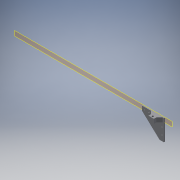
# Autodesk Inventor part: Bed Bracket
Saved by Autodesk Inventor 2016 (Build 200138000, 138)
## iProperties
Created: 2016-05-26
Part Number: Bed Bracket
Material: Generic
Document SubType Name: Modeling
Designer: Scott
Density: 1 g/cm^3
Appearance: Default
Author: Scott
Autodesk Inventor part; units mm, degrees
ref_plane "YZ Plane" through (0, 0, 0) normal (1, 0, 0) x (0, 1, 0)
ref_plane "XZ Plane" through (0, 0, 0) normal (0, 1, 0) x (-1, 0, 0)
ref_plane "XY Plane" through (0, 0, 0) normal (0, 0, 1) x (1, 0, 0)
ref_plane "Work Plane1" through (0, 0, 0) normal (0, 0, 1) x (1, 0, 0)
sketch "Sketch1" plane through (0, 0, 0) normal (0, 0, 1) x (1, 0, 0)
  line L0 (0, 0) -> (304.8, 0)
  line L1 (304.8, 0) -> (292.1, 0)
  line L2 (-330.2, 20) -> (330.2, 20) projected
  line L3 (-330.2, 0) -> (-330.2, 20) projected
  line L4 (330.2, 0) -> (-330.2, 0) projected
  line L5 (330.2, 20) -> (330.2, 0) projected
  line L6 (292.1, 0) -> (292.1, 10)
  line L7 (330.6445, 0) -> (253.5555, 0)
  line L8 (253.5555, 0) -> (253.5555, 20)
  line L9 (253.5555, 20) -> (330.6445, 20)
  line L10 (330.6445, 20) -> (330.6445, 0)
  line L11 (330.6445, 0) -> (253.5555, 20) construction
  line L12 (253.5555, 0) -> (330.6445, 20) construction
  line L13 (330.6445, 0) -> (330.6445, -76.2)
  line L14 (330.6445, 0) -> (406.8445, 0) construction
  line L15 (330.6445, -76.2) -> (310.8751, -76.2)
  line L16 (330.6445, 20) -> (229.0445, 20)
  line L17 (229.0445, 20) -> (229.0445, 0)
  line L18 (229.0445, 0) -> (310.8751, -76.2)
  line L19 (310.8751, -76.2) -> (310.8751, 0)
  dimension "d0" = 304.8
  dimension "d1" = 12.7
  dimension "d2" = 76.2
  dimension "d3" = 90
  dimension "d4" = 101.6
  constraints: 32 end point, 5 point on line, 4 parallel, 3 horizontal, 3 perpendicular, 2 midpoint, 2 vertical
  measures "d0" distance of L0.start L0.end
  measures "d1" distance of L0.end L1.end
  measures "d2" distance of L7.start L13.end
  measures "d3" angle of L13 L14
  measures "d4" distance of L9.end L16.end
extrude "Extrusion1" add sketch "Sketch1" along normal blind 5.08 contours L17 L2 L8 L0 | L0 L4 L19 L18 | L8 L2 L5 L4 L0 | L19 L4 L7 L13 L15 | L9 L10 L7 L5
sketch "Sketch2" plane through (0, 0, 5.08) normal (0, 0, 1) x (1, 0, 0)
  line L0 (310.2, -876.3) -> (310.2, 0) projected
  line L1 (310.2, 0) -> (297.5, 0)
  line L2 (297.5, 0) -> (297.5, 10)
  line L3 (284.8, 20) -> (310.2, 20)
  line L4 (310.2, 20) -> (310.2, 0)
  line L5 (310.2, 0) -> (284.8, 0)
  line L6 (284.8, 0) -> (284.8, 20)
  line L7 (284.8, 20) -> (310.2, 0) construction
  line L8 (310.2, 20) -> (284.8, 0) construction
  point P0 (0, 0)
  dimension "d7" = 12.7
  dimension "d8" = 10
  dimension "d9" = 90
  constraints: 16 end point, 2 horizontal, 2 midpoint, 2 parallel, 2 perpendicular
  measures "d7" distance of L0.end L1.end
  measures "d8" distance of L1.end L2.end
  measures "d9" angle of L1 L2
extrude "Extrusion2" add sketch "Sketch2" along normal blind 25.4
sketch "Sketch3" plane through (229.0445, 20, 0) normal (0, 1, 0) x (1, 0, 0)
  line L0 (101.6, 0) -> (0, 0) projected
  line L1 (0, 0) -> (0, -5.08) projected
  line L2 (55.7555, -5.08) -> (0, -5.08) projected
  line L3 (55.7555, -5.08) -> (55.7555, -30.48) projected
  line L4 (81.1555, -30.48) -> (55.7555, -30.48) projected
  line L5 (81.1555, -5.08) -> (81.1555, -30.48) projected
  line L6 (101.6, -5.08) -> (81.1555, -5.08) projected
  line L7 (101.6, 0) -> (101.6, -5.08) projected
  circle A0 centre (68.4555, -22.86) radius 4
  point P0 (-229.0445, 0)
  dimension "d12" = 8
  dimension "d13" = 7.62
  constraints: 1 centre point
  measures "d12" diameter of A0
  measures "d13" distance from line of L4 A0.centre
extrude "Extrusion3" cut sketch "Sketch3" against normal blind 101.6 contours A0
chamfer "Chamfer1" distance 14.2875 angle 45 2 edges at (284.8, 10, 5.08) (310.2, 10, 5.08)
sketch "Sketch4" plane through (0, 0, 5.08) normal (0, 0, 1) x (1, 0, 0)
  line L0 (324.4875, 0) -> (324.4875, 20) projected
  line L1 (324.4875, 0) -> (270.5125, 0) projected
  line L2 (270.5125, 20) -> (270.5125, 0) projected
  line L3 (270.5125, 20) -> (229.0445, 20) projected
  line L4 (229.0445, 20) -> (229.0445, 0) projected
  line L5 (229.0445, 0) -> (310.8751, -76.2) projected
  line L6 (310.8751, -76.2) -> (330.6445, -76.2) projected
  line L7 (330.6445, -76.2) -> (330.6445, 20) projected
  line L8 (330.6445, 20) -> (324.4875, 20) projected
  line L9 (330.2, 0) -> (330.2, -876.3) projected
  line L10 (310.2, 0) -> (330.2, 0) projected
  line L11 (310.2, -876.3) -> (310.2, 0) projected
  line L12 (330.2, -876.3) -> (310.2, -876.3) projected
  line L13 (324.4875, 0) -> (324.4875, 20) projected
  line L14 (324.4875, 0) -> (270.5125, 0) projected
  line L15 (270.5125, 20) -> (270.5125, 0) projected
  line L16 (270.5125, 20) -> (229.0445, 20) projected
  line L17 (229.0445, 20) -> (229.0445, 0) projected
  line L18 (229.0445, 0) -> (310.8751, -76.2) projected
  line L19 (310.8751, -76.2) -> (330.6445, -76.2) projected
  line L20 (330.6445, -76.2) -> (330.6445, 20) projected
  line L21 (330.6445, 20) -> (324.4875, 20) projected
  line L22 (330.2, 0) -> (-330.2, 0) projected
  circle A0 centre (320.7598, -50.8) radius 2.5
  circle A1 centre (320.7598, -19.05) radius 2.5
  circle A2 centre (241.7445, 10) radius 2.5
  circle A3 centre (260.7945, 10) radius 2.5
  point P0 (0, 0)
  dimension "d19" = 5
  dimension "d20" = 5
  dimension "d21" = 31.75
  dimension "d22" = 25.4
  dimension "d23" = 5
  dimension "d24" = 5
  dimension "d25" = 12.7
  dimension "d26" = 19.05
  constraints: 4 centre point
  measures "d19" diameter of A0
  measures "d20" diameter of A1
  measures "d21" distance of A0.centre A1.centre
  measures "d22" distance from line of L6 A0.centre
  measures "d23" diameter of A2
  measures "d24" diameter of A3
  measures "d25" distance from line of L4 A2.centre
  measures "d26" distance of A2.centre A3.centre
extrude "Extrusion4" cut sketch "Sketch4" against normal blind 101.6 contours A0 | A1 | A2 | A3
body "Solid1"
